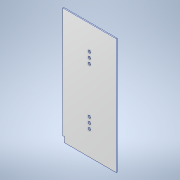
# Autodesk Inventor part: 7001_Aluminum_Chasis_Coil_Assembly_Separator_Tx_Filter_MPSv2_v1
Saved by Autodesk Inventor 2021 (Build 250183000, 183)
## iProperties
Created: 2020-11-18
Part Number: 7001_Aluminum_Chasis_Coil_Assembly_Separator_Tx_Filter_MPSv2_v1
Material: Aluminum 6061
Document SubType Name: Modeling
Designer: Admin
Density: 2.7 g/cm^3
Appearance: Aluminum - Flat
Author: Admin
Autodesk Inventor part; units mm, degrees
ref_plane "YZ Plane" through (0, 0, 0) normal (1, 0, 0) x (0, 1, 0)
ref_plane "XZ Plane" through (0, 0, 0) normal (0, 1, 0) x (-1, 0, 0)
ref_plane "XY Plane" through (0, 0, 0) normal (0, 0, 1) x (1, 0, 0)
sketch "Sketch1" plane through (0, 0, 0) normal (0, 0, 1) x (1, 0, 0)
  line L0 (0, 0) -> (101.5, 0)
  line L1 (101.5, 0) -> (101.5, -220)
  line L2 (101.5, -220) -> (0, -220)
  line L3 (0, -220) -> (0, 0)
  dimension "d0" = 101.5
  dimension "d1" = 220
  constraints: 8 end point, 2 parallel, 1 horizontal, 1 perpendicular
  measures "d0" distance of L1.end L2.end
  measures "d1" distance of L0.end L1.end
extrude "Extrusion1" add sketch "Sketch1" along normal blind 1.8
sketch "Sketch2" plane through (0, 0, 1.8) normal (0, 0, 1) x (1, 0, 0)
  line L0 (0, 0) -> (0, -220) projected
  line L1 (101.5, -220) -> (101.5, 0) projected
  line L2 (0, 0) -> (101.5, 0)
  line L3 (101.5, 0) -> (101.5, -10)
  line L4 (101.5, -10) -> (0, -10)
  line L5 (0, -10) -> (0, 0)
  line L6 (50.75, -10) -> (140.75, -10)
  line L7 (140.75, -10) -> (140.75, -153.5958)
  line L8 (140.75, -153.5958) -> (50.75, -153.5958)
  line L9 (50.75, -153.5958) -> (50.75, -10)
  circle A0 centre (50.75, -153.5958) radius 2.5
  line L10 (50.75, -153.5958) -> (50.75, -173.5958)
  circle A1 centre (50.75, -173.5958) radius 2.5
  line L11 (50.75, -153.5958) -> (50.75, -133.5958)
  circle A2 centre (50.75, -163.5958) radius 2.5
  line L12 (101.5, 0) -> (0, 0) projected
  line L13 (0, -220) -> (101.5, -220) projected
  line L14 (0, 0) -> (101.5, -220)
  line L15 (101.5, -220) -> (50.75, -110)
  line L16 (50.75, -110) -> (87.135, -110)
  circle A3 centre (50.75, -66.4042) radius 2.5
  line L17 (50.75, -113.5958) -> (50.75, -46.4042)
  circle A4 centre (50.75, -46.4042) radius 2.5
  line L18 (50.75, -113.5958) -> (50.75, -86.4042)
  circle A5 centre (50.75, -56.4042) radius 2.5
  dimension "d4" = 10
  dimension "d5" = 90
  dimension "d6" = 5
  dimension "d7" = 20
  dimension "d8" = 20
  dimension "d11" = 5
  constraints: 30 end point, 6 centre point, 4 coincident, 4 parallel, 3 horizontal, 3 midpoint, 2 perpendicular, 2 point on line, 2 symmetric about line, 1 vertical
  measures "d4" distance of L2.end L3.end
  measures "d5" distance of L7.end L8.end
  measures "d6" diameter of A0
  measures "d7" distance of L10.start L10.end
  measures "d8" distance of L10.start L11.end
  measures "d11" diameter of A2
extrude "Extrusion2" cut sketch "Sketch2" against normal blind 10 contours A4 L9 | L9 A4 | A3 L9 | L9 A3 | A0 L10 L8 | L8 L9 A0 | A5 L9 | L9 A5 | L9 L10 A0 | A2 L10 | L10 A2 | A1
sketch "Sketch3" plane through (0, 0, 1.8) normal (0, 0, 1) x (1, 0, 0)
  line L0 (0, -220) -> (101.5, -220) projected
  line L1 (0, -220) -> (3, -220)
  line L2 (3, -220) -> (3, -210)
  line L3 (3, -210) -> (0, -210)
  line L4 (0, -210) -> (0, -220)
  point P0 (0, 0)
  dimension "d14" = 3
  dimension "d15" = 10
  constraints: 8 end point, 2 parallel, 1 horizontal, 1 perpendicular
  measures "d14" distance of L3.end L2.end
  measures "d15" distance of L2.end L1.end
extrude "Extrusion3" cut sketch "Sketch3" against normal blind 10
body "Solid1"
